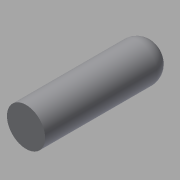
# Autodesk Inventor part: plastik kafa
Saved by Autodesk Inventor 2017 (Build 210142000, 142)
## iProperties
Created: 2017-03-16
Part Number: plastik kafa
Material: Generic
Document SubType Name: Modeling
Designer: Win10
Density: 1 g/cm^3
Appearance: Default
Author: Win10
Autodesk Inventor part; units mm, degrees
ref_plane "YZ Plane" through (0, 0, 0) normal (1, 0, 0) x (0, 1, 0)
ref_plane "XZ Plane" through (0, 0, 0) normal (0, 1, 0) x (-1, 0, 0)
ref_plane "XY Plane" through (0, 0, 0) normal (0, 0, 1) x (1, 0, 0)
sketch "Sketch1" plane through (0, 0, 0) normal (0, 1, 0) x (-1, 0, 0)
  circle A0 centre (0, 0) radius 1.875 construction
  circle A1 centre (0, 0) radius 1.495
  dimension "d0" = 3.75
  dimension "d1" = 0.38
  constraints: 2 centre point, 1 coincident
  measures "d0" diameter of A0
  measures "d1" radial gap between concentric circles of A0 A1
extrude "Extrusion1" add sketch "Sketch1" along normal blind 8.5
fillet "Fillet1" radius 1.25 1 edges at (1.495, 8.5, 0)
body "Solid1"
